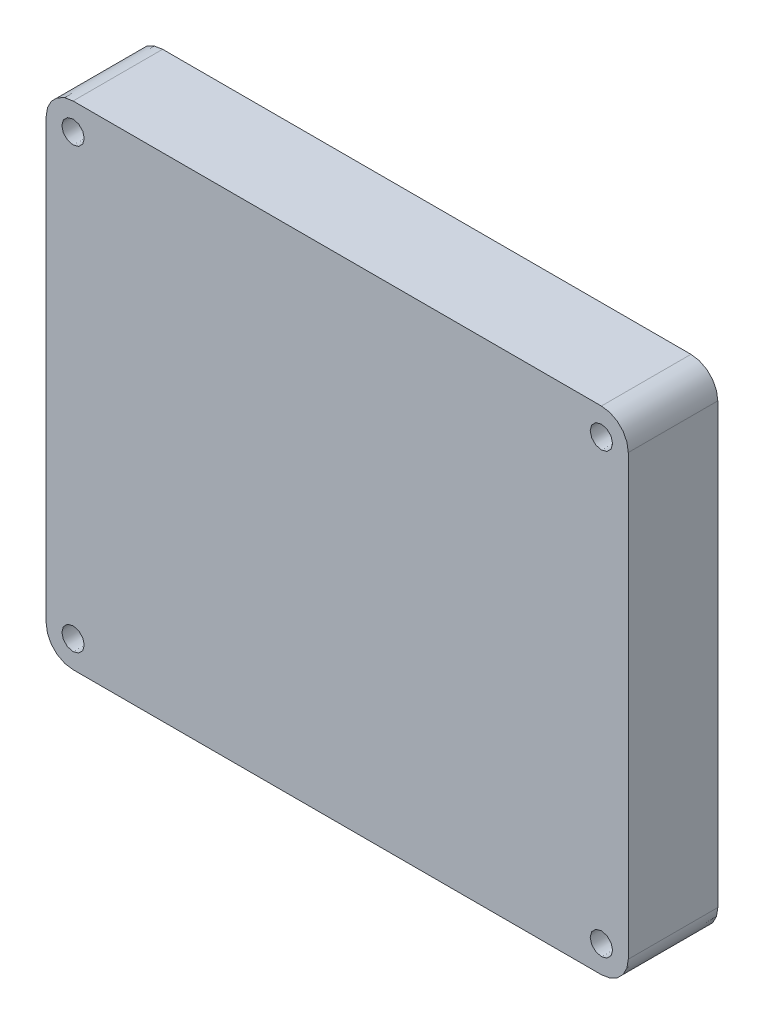
# Autodesk Inventor part: header
Saved by Autodesk Inventor 2017.2 (Build 212233000, 233)
## iProperties
Created: 2017-09-05
Part Number: header
Material: Generic
Document SubType Name: Modeling
Designer: Nic
Density: 1 g/cm^3
Appearance: Default
Author: Nic
Autodesk Inventor part; units mm, degrees
ref_plane "YZ Plane" through (0, 0, 0) normal (1, 0, 0) x (0, 1, 0)
ref_plane "XZ Plane" through (0, 0, 0) normal (0, 1, 0) x (-1, 0, 0)
ref_plane "XY Plane" through (0, 0, 0) normal (0, 0, 1) x (1, 0, 0)
sketch "Sketch1" plane through (0, 0, 0) normal (0, 0, 1) x (1, 0, 0)
  line L0 (-29.5, 27.5) -> (29.5, 27.5)
  line L1 (32.5, 24.5) -> (32.5, -24.5)
  line L2 (29.5, -27.5) -> (-29.5, -27.5)
  line L3 (-32.5, -24.5) -> (-32.5, 24.5)
  line L4 (0, 0) -> (32.5, 0) construction
  line L5 (0, 0) -> (0, 27.5) construction
  arc A0 (-32.5, -24.5) -> (-29.5, -27.5) centre (-29.5, -24.5) ccw
  arc A1 (-29.5, 27.5) -> (-32.5, 24.5) centre (-29.5, 24.5) ccw
  arc A2 (32.5, 24.5) -> (29.5, 27.5) centre (29.5, 24.5) ccw
  arc A3 (29.5, -27.5) -> (32.5, -24.5) centre (29.5, -24.5) ccw
  circle A4 centre (-29.5, -24.5) radius 1.25
  circle A5 centre (-29.5, 24.5) radius 1.25
  circle A6 centre (29.5, -24.5) radius 1.25
  circle A7 centre (29.5, 24.5) radius 1.25
  point P0 (-32.5, 27.5)
  point P1 (32.5, -27.5)
  point P2 (32.5, 27.5)
  point P3 (-32.5, -27.5)
  dimension "d1" = 65
  dimension "d5" = 3
  dimension "d6" = 2.5
  dimension "d9" = 49
  constraints: 12 end point, 8 centre point, 8 point on circle, 8 point on line, 8 tangent, 3 equal radius, 3 symmetric about line, 2 horizontal, 2 midpoint, 2 parallel, 2 perpendicular, 1 concentric, 5 other
  measures "d1" distance of point (32.5, -27.5) point (-32.5, -27.5)
  measures "d5" radius of A1
  measures "d6" diameter of A4
  measures "d9" distance of A2.centre A3.centre
extrude "Extrusion1" add sketch "Sketch1" along normal blind 10
body "Solid1"
